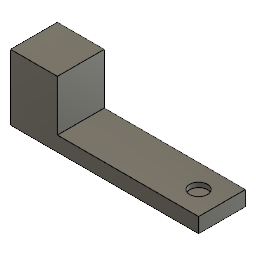
Untitled v2 (Autodesk Fusion 360 design; units mm, degrees)
Autodesk Fusion 360 part; units mm, degrees
note: some values were not read from the file. Set by a fixed rule: which sketch regions a step uses.
sketch "Sketch2" plane through (0, 0, 0) normal (0, 1, 0) x (1, 0, 0) in component "tabs"
  line L0 (0, 0) -> (30, 0)
  line L1 (30, 0) -> (30, 10)
  line L2 (30, 10) -> (0, 10)
  line L3 (0, 10) -> (0, 0)
  dimension "d5" = 30
  measures "d5" distance of L0.start L0.end
sketch "Sketch1" plane through (0, 0, 0) normal (0, 1, 0) x (1, 0, 0) in component "tabs"
  line L0 (-10, 0) -> (0, 0)
  line L1 (0, 0) -> (0, 10)
  line L2 (0, 10) -> (-10, 10)
  line L3 (-10, 10) -> (-10, 0)
  dimension "d1" = 10
  dimension "d2" = 10
  measures "d1" distance of L0.start L0.end
  measures "d2" distance of L0.start L2.end
extrude "Extrude1" add sketch "Sketch1" along normal blind 14 in component "tabs"
extrude "Extrude2" add sketch "Sketch2" along normal blind 3.2 in component "tabs"
sketch "Sketch3" plane through (0, 3.2, 0) normal (0, 1, 0) x (-1, 0, 0) in component "tabs"
  line L0 (0, -10) -> (0, 0)
  line L1 (0, 0) -> (-30, 0)
  line L2 (-30, 0) -> (-30, -10)
  line L3 (-30, -10) -> (0, -10)
  line L4 (-30, -5) -> (-25, -5) construction
  circle A0 centre (-25, -5) radius 1.9
  line L5 (0, -5) -> (-26.2356, -5) construction
  dimension "d8" = 3.8
  measures "d8" diameter of A0
extrude "Extrude3" cut sketch "Sketch3" against normal blind 1 contours A0 in component "tabs"
component "tabs" placed x (1, 0, 0) y (0, 1, 0) z (0, 0, 1) at (0, 0, 0)
